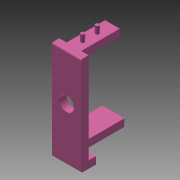
# Autodesk Inventor part: Spool Holder Cap Section Mk1
Saved by Autodesk Inventor 2015 (Build 190159000, 159)
## iProperties
Created: 2016-11-23
Part Number: Spool Holder Cap Section Mk1
Material: Generic
Document SubType Name: Modeling
Designer: Markus
Density: 1 g/cm^3
Appearance: Pink
Author: Markus
Autodesk Inventor part; units mm, degrees
ref_plane "YZ Plane" through (0, 0, 0) normal (1, 0, 0) x (0, 1, 0)
ref_plane "XZ Plane" through (0, 0, 0) normal (0, 1, 0) x (-1, 0, 0)
ref_plane "XY Plane" through (0, 0, 0) normal (0, 0, 1) x (1, 0, 0)
sketch "Sketch1" plane through (0, 0, 0) normal (0, 0, 1) x (1, 0, 0)
  line L0 (0, 0) -> (12.7, 0)
  line L1 (12.7, 0) -> (12.7, 6.35)
  line L2 (12.7, 6.35) -> (0, 6.35)
  line L3 (0, 6.35) -> (0, 0)
  line L4 (-3.175, -59.7408) -> (15.875, -59.7408)
  line L5 (15.875, -59.7408) -> (15.875, -66.0908)
  line L6 (15.875, -66.0908) -> (-3.175, -66.0908)
  line L7 (-3.175, -66.0908) -> (-3.175, -59.7408)
  line L8 (-9.525, -59.7408) -> (22.225, -59.7408) construction
  line L9 (15.875, -59.7408) -> (-3.175, -66.0908) construction
  line L10 (-3.175, -59.7408) -> (15.875, -66.0908) construction
  line L11 (6.35, -62.9158) -> (15.875, -62.9158) construction
  point P0 (6.35, 6.35)
  point P1 (6.35, -59.7408)
  dimension "d0" = 12.7
  dimension "d1" = 6.35
  dimension "d2" = 6.35
  dimension "d3" = 31.75
  dimension "d4" = 69.2658
  dimension "d5" = 6.35
  dimension "d6" = 6.35
  constraints: 24 end point, 5 midpoint, 4 parallel, 3 horizontal, 2 perpendicular, 1 vertical alignment
  measures "d0" distance of L1.end L2.end
  measures "d1" distance of L2.end L0.start
  measures "d2" distance of L4.end L5.end
  measures "d3" distance of L8.start L8.end
  measures "d4" distance from line of L2 L11.end
  measures "d5" distance from line of L8.start L7
  measures "d6" distance from line of L8.end L5
extrude "Extrusion1" add sketch "Sketch1" along normal blind 34.29
sketch "Sketch2" plane through (0, 0, 34.29) normal (0, 0, 1) x (1, 0, 0)
  line L0 (-6.35, 6.35) -> (19.05, 6.35)
  line L1 (19.05, 6.35) -> (19.05, -78.8924)
  line L2 (19.05, -78.8924) -> (-6.35, -78.8924)
  line L3 (-6.35, -78.8924) -> (-6.35, 6.35)
  line L4 (0, 0) -> (12.7, 0) projected
  line L5 (12.7, 0) -> (12.7, 6.35) projected
  line L6 (12.7, 6.35) -> (0, 6.35) projected
  line L7 (0, 6.35) -> (0, 0) projected
  point P0 (6.35, 6.35)
  point P1 (6.35, 6.35)
  dimension "d9" = 25.4
  dimension "d10" = 85.2424
  constraints: 8 end point, 2 midpoint, 2 parallel, 1 coincident, 1 horizontal, 1 horizontal alignment, 1 perpendicular, 1 point on line
  measures "d9" distance between parallel lines of L1 L3
  measures "d10" distance of L2.end L0.start
extrude "Extrusion2" add sketch "Sketch2" along normal blind 6.35
sketch "Sketch3" plane through (0, 0, 34.29) normal (0, 0, -1) x (-1, 0, 0)
  line L0 (-15.875, -66.0908) -> (-15.875, -59.7408) projected
  line L1 (-15.875, -59.7408) -> (3.175, -59.7408) projected
  line L2 (3.175, -59.7408) -> (3.175, -66.0908) projected
  line L3 (3.175, -66.0908) -> (-15.875, -66.0908) projected
  line L4 (-12.7, 0) -> (-12.7, 6.35) projected
  line L5 (-12.7, 6.35) -> (-19.05, 6.35) projected
  line L6 (-19.05, 6.35) -> (-19.05, -78.8924) projected
  line L7 (-19.05, -78.8924) -> (6.35, -78.8924) projected
  line L8 (6.35, -78.8924) -> (6.35, 6.35) projected
  line L9 (6.35, 6.35) -> (0, 6.35) projected
  line L10 (0, 6.35) -> (0, 0) projected
  line L11 (0, 0) -> (-12.7, 0) projected
  line L12 (6.35, 6.35) -> (6.35, -78.8924) projected
  line L13 (-19.05, -78.8924) -> (6.35, -78.8924)
  line L14 (6.35, -78.8924) -> (6.35, -72.5424)
  line L15 (6.35, -72.5424) -> (-19.05, -72.5424)
  line L16 (-19.05, -72.5424) -> (-19.05, -78.8924)
  dimension "d13" = 6.35
  constraints: 8 end point, 2 parallel, 1 horizontal, 1 perpendicular, 1 point on line
  measures "d13" distance between parallel lines of L7 L15
extrude "Extrusion3" add sketch "Sketch3" along normal blind 6.35 contours L15 L8 L7 L6
sketch "Sketch4" plane through (0, 6.35, 0) normal (0, 1, 0) x (1, 0, 0)
  line L0 (12.7, 0) -> (0, 0) projected
  line L1 (0, 0) -> (0, -34.29) projected
  line L2 (-6.35, -34.29) -> (0, -34.29) projected
  line L3 (-6.35, -34.29) -> (-6.35, -40.64) projected
  line L4 (19.05, -40.64) -> (-6.35, -40.64) projected
  line L5 (19.05, -34.29) -> (19.05, -40.64) projected
  line L6 (12.7, -34.29) -> (19.05, -34.29) projected
  line L7 (12.7, 0) -> (12.7, -34.29) projected
  line L8 (15.875, 0) -> (-3.175, 0) construction
  line L9 (6.35, 0) -> (6.35, -40.64) construction
  line L10 (-6.35, -40.64) -> (19.05, -40.64) construction
  line L11 (0, -34.29) -> (0, -40.64) construction
  line L12 (12.7, -34.29) -> (12.7, -40.64) construction
  line L13 (12.7, -40.64) -> (0, 0) construction
  line L14 (0, -40.64) -> (12.7, 0) construction
  circle A0 centre (6.35, -26.67) radius 1.5875
  circle A1 centre (6.35, -13.97) radius 1.5875
  line L15 (6.35, -20.32) -> (0, -20.32) construction
  point P0 (0, 0)
  dimension "d16" = 3.175
  dimension "d17" = 6.35
  dimension "d18" = 6.35
  constraints: 12 end point, 5 point on line, 3 midpoint, 2 centre point, 2 perpendicular, 1 equal radius, 1 vertical
  measures "d16" diameter of A0
  measures "d17" distance from line of L15 A0.centre
  measures "d18" distance of A1.centre L15.start
extrude "Extrusion4" add sketch "Sketch4" along normal blind 6.35 contours A0 | A1
sketch "Sketch5" plane through (0, 0, 40.64) normal (0, 0, 1) x (1, 0, 0)
  line L0 (19.05, 6.35) -> (-6.35, 6.35) projected
  line L1 (-6.35, 6.35) -> (-6.35, -78.8924) projected
  line L2 (-6.35, -78.8924) -> (19.05, -78.8924) projected
  line L3 (19.05, -78.8924) -> (19.05, 6.35) projected
  circle A0 centre (6.35, -33.02) radius 6.3881
  point P0 (0, 0)
  point P1 (6.35, 6.35)
  dimension "d21" = 12.7762
  dimension "d22" = 39.37
  constraints: 1 centre point, 1 midpoint, 1 vertical alignment
  measures "d21" diameter of A0
  measures "d22" distance from line of L0 A0.centre
extrude "Extrusion5" cut sketch "Sketch5" against normal up to surface (6.35 mm away) contours A0
fillet "Fillet2" radius 1.27 3 edges at (6.35, 6.35, 40.64) (6.35, -78.8924, 40.64) (6.35, 6.35, 0)
equation "\"d6\" = d5"
equation "\"d18\" = d17"
body "Solid1"
